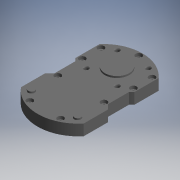
# Autodesk Inventor part: Gehaeusedeckel_Parallelform
Saved by Autodesk Inventor 2017.3 (Build 213256000, 256)
## iProperties
Part Number: Gehaeusedeckel_Parallelform
Material: Generic
Catalog Web Link: www.cadenas.de
Description: Geheausedecke-Bauteil LZ80
Vendor: ROSEKRIEGER
Document SubType Name: Modeling
Designer: partserver
Manufacturer: ROSEKRIEGER
Mass: 369.888 g
Surface Area: 551.39 cm^2
Volume: 369.888 cm^3
Density: 1 g/cm^3
Appearance: PSOLRGB-128-128-128
Category: PARTsolutions
Company: ROSEKRIEGER
Title: Gehaeusedeckel_Parallelform
Author: Cadenas PARTsolutions
Comments: Bauteil LZ80
PSOL_IDENT_0: {$CADENAS_DATA\23d-libs\rose_krieger\linearkomponenten\pool_lineartechnik\_hubsaeule_zyliinder\elekt
PSOL_IDENT_1: rozylinder\elekzyl_lz80\lz80_gehaeusedeckel.prj},192 {VTYP=3D},{NB=Gehaeusedeckel_Parallelform},{LIN
PSOL_IDENT_2: A=Gehaeusedeckel_Parallelform},{NN=Geheausedecke},{DATE=12.11.2020 14:43:35},{GEOMDATE=06.12.2006},{
PSOL_IDENT_3: VERSION=},{LINEID=10},{WBVAR=},{WBNUMERIC=}  {NB=Gehaeusedeckel_Parallelform},{LINA=Gehaeusedeckel_P
PSOL_IDENT_4: arallelform},{KT=DUMMY},{IDNR=},{ARTIKEL=Gehaeusedeckel_Parallelform},{DECKELBR1=107.310},{DECKELBR2=
PSOL_IDENT_5: 114.310},{DECKELBR3=97.310},{KONTRA1=71.450},{KONTRA2=74.100},{ABKONTRA2=25.250},{ABKONTRA1=25.240},
PSOL_IDENT_6: {ACHSAB=95.760},{HOEHE=20.000},{FUSSGROSS=44.500},{FUSSKLEIN=12.000},{FUSSKLHOE=3.000},{FUSSGRHOE=3.
PSOL_IDENT_7: 000},{ABFUSKL=18.000},{BREITFUSKL=84.000},{BEFBO1=7.450},{ABBEFBO1=56.500},{TIEFBEFBO1=20.500},{SENK
PSOL_IDENT_8: DURCH=9.500},{FASE=1.500},{SENKDURCH1=11.200},{SENKDURCH2=6.400},{SENKTIEF1=5.500},{ABSENK3U4=93.000
PSOL_IDENT_9: },{ABSENK1=84.000},{ABSENK2=56.000},{ABSENK5=39.500},{SENKAB4=113.000},{SENKAB3=79.000},{SENKAB1=30.
PSOL_IDENT_10: 000},{SENKAB2=35.000}
NB: Gehaeusedeckel_Parallelform
NN: Geheausedecke
NT: Bauteil LZ80
NBSYN: $ARTIKEL.
LINA: Gehaeusedeckel_Parallelform
CATALOG: RK Rose+Krieger
ARTIKEL: Gehaeusedeckel_Parallelform
DECKELBR1: 107.31
DECKELBR2: 114.31
DECKELBR3: 97.31
KONTRA1: 71.45
KONTRA2: 74.1
ABKONTRA2: 25.25
ABKONTRA1: 25.24
ACHSAB: 95.76
HOEHE: 20
FUSSGROSS: 44.5
FUSSKLEIN: 12
FUSSKLHOE: 3
FUSSGRHOE: 3
ABFUSKL: 18
BREITFUSKL: 84
BEFBO1: 7.45
ABBEFBO1: 56.5
TIEFBEFBO1: 20.5
SENKDURCH: 9.5
FASE: 1.5
SENKDURCH1: 11.2
SENKDURCH2: 6.4
SENKTIEF1: 5.5
ABSENK3U4: 93
ABSENK1: 84
ABSENK2: 56
ABSENK5: 39.5
SENKAB4: 113
SENKAB3: 79
SENKAB1: 30
SENKAB2: 35
SUPPLIER: ROSEKRIEGER
ARTICLENO: Gehaeusedeckel_Parallelform
BOMINFO: Gehaeusedeckel_Parallelform
CREATOR: CADENAS GmbH
Autodesk Inventor part; units mm, degrees
ref_plane "YZ Plane" through (0, 0, 0) normal (1, 0, 0) x (0, 1, 0)
ref_plane "XZ Plane" through (0, 0, 0) normal (0, 1, 0) x (-1, 0, 0)
ref_plane "XY Plane" through (0, 0, 0) normal (0, 0, 1) x (1, 0, 0)
sketch "Skizze_1" plane through (0, 0, 0) normal (0, 0, 1) x (1, 0, 0)
  line L0 (-57.155, -25.9695) -> (-57.155, -69.7905)
  arc A0 (-57.155, -69.7905) -> (57.155, -69.7905) centre (0, -22.63) ccw
  line L1 (57.155, -69.7905) -> (57.155, -25.9695)
  arc A1 (57.155, -25.9695) -> (48.655, -17.2417) centre (0, -73.13) ccw
  line L2 (48.655, -17.2417) -> (48.655, 20.7961)
  arc A2 (48.655, 20.7961) -> (53.655, 25.9369) centre (0, 73.12) ccw
  line L3 (53.655, 25.9369) -> (53.655, 69.8231)
  arc A3 (53.655, 69.8231) -> (-53.655, 69.8231) centre (0, 22.64) ccw
  line L4 (-53.655, 69.8231) -> (-53.655, 25.9369)
  arc A4 (-53.655, 25.9369) -> (-48.655, 20.7961) centre (0, 73.12) ccw
  line L5 (-48.655, 20.7961) -> (-48.655, -17.2417)
  arc A5 (-48.655, -17.2417) -> (-57.155, -25.9695) centre (0, -73.13) ccw
  constraints: 12 end point, 12 point on circle, 6 centre point
extrude "Extrusion1" add sketch "Skizze_1" along normal blind 20
sketch "Skizze_2" plane through (0, 0, 0) normal (0, 0, 1) x (1, 0, 0)
  circle A0 centre (0, 47.88) radius 22.25
  constraints: 1 centre point
extrude "Extrusion2" add sketch "Skizze_2" against normal blind 3
sketch "Skizze_3" plane through (0, 0, 0) normal (0, 0, 1) x (1, 0, 0)
  circle A0 centre (42, -65.88) radius 6
  constraints: 1 centre point
extrude "Extrusion3" add sketch "Skizze_3" against normal blind 3
sketch "Skizze_4" plane through (0, 0, 0) normal (0, 0, 1) x (1, 0, 0)
  circle A0 centre (-42, -65.88) radius 6
  constraints: 1 centre point
extrude "Extrusion4" add sketch "Skizze_4" against normal blind 3
sketch "Skizze_6" plane through (0, 0, 20) normal (0, 0, 1) x (1, 0, 0)
  circle A0 centre (28.25, 76.13) radius 4.75
  constraints: 1 centre point
extrude "Extrusion5" add sketch "Skizze_6" along normal blind 3
pattern_linear "Rectangular Pattern1" count 2 spacing 56.5 along (-1, 0, 0) count 2 spacing 56.5 along (0, -1, 0) of "Extrusion5"
sketch "Sketch6" plane through (0, 0, 0) normal (0, 0, -1) x (-1, 0, 0)
  point P0 (-28.25, 19.63)
hole "Hole1" at (28.25, 19.63, 0) direction (0, 0, 1) diameter 7.45 depth 20.5 countersink diameter 9.5 countersink angle 68.692
sketch "Sketch7" plane through (0, 0, 0) normal (0, 0, -1) x (-1, 0, 0)
  point P0 (-28.25, 76.13)
hole "Hole2" at (28.25, 76.13, 0) direction (0, 0, 1) diameter 7.45 depth 20.5 countersink diameter 9.5 countersink angle 68.692
sketch "Sketch8" plane through (0, 0, 0) normal (0, 0, -1) x (-1, 0, 0)
  point P0 (28.25, 19.63)
hole "Hole3" at (-28.25, 19.63, 0) direction (0, 0, 1) diameter 7.45 depth 20.5 countersink diameter 9.5 countersink angle 68.692
sketch "Sketch9" plane through (0, 0, 0) normal (0, 0, -1) x (-1, 0, 0)
  point P0 (28.25, 76.13)
hole "Hole4" at (-28.25, 76.13, 0) direction (0, 0, 1) diameter 7.45 depth 20.5 countersink diameter 9.5 countersink angle 68.692
sketch "Sketch10" plane through (0, 0, 0) normal (0, 0, -1) x (-1, 0, 0)
  point P0 (0, 87.38)
hole "Hole5" at (0, 87.38, 0) direction (0, 0, 1) diameter 6.4 depth 20 counterbore diameter 11.2 counterbore depth 5.5
sketch "Sketch11" plane through (0, 0, 0) normal (0, 0, -1) x (-1, 0, 0)
  point P0 (46.5, 65.12)
hole "Hole6" at (-46.5, 65.12, 0) direction (0, 0, 1) diameter 6.4 depth 20 counterbore diameter 11.2 counterbore depth 5.5
sketch "Sketch12" plane through (0, 0, 0) normal (0, 0, -1) x (-1, 0, 0)
  point P0 (46.5, 31.12)
hole "Hole7" at (-46.5, 31.12, 0) direction (0, 0, 1) diameter 6.4 depth 20 counterbore diameter 11.2 counterbore depth 5.5
sketch "Sketch13" plane through (0, 0, 0) normal (0, 0, -1) x (-1, 0, 0)
  point P0 (42, -17.88)
hole "Hole8" at (-42, -17.88, 0) direction (0, 0, 1) diameter 6.4 depth 20 counterbore diameter 11.2 counterbore depth 5.5
sketch "Sketch14" plane through (0, 0, 0) normal (0, 0, -1) x (-1, 0, 0)
  point P0 (28, -82.88)
hole "Hole9" at (-28, -82.88, 0) direction (0, 0, 1) diameter 6.4 depth 20 counterbore diameter 11.2 counterbore depth 5.5
sketch "Sketch15" plane through (0, 0, 0) normal (0, 0, -1) x (-1, 0, 0)
  point P0 (-46.5, 65.12)
hole "Hole10" at (46.5, 65.12, 0) direction (0, 0, 1) diameter 6.4 depth 20 counterbore diameter 11.2 counterbore depth 5.5
sketch "Sketch16" plane through (0, 0, 0) normal (0, 0, -1) x (-1, 0, 0)
  point P0 (-46.5, 31.12)
hole "Hole11" at (46.5, 31.12, 0) direction (0, 0, 1) diameter 6.4 depth 20 counterbore diameter 11.2 counterbore depth 5.5
sketch "Sketch17" plane through (0, 0, 0) normal (0, 0, -1) x (-1, 0, 0)
  point P0 (-42, -17.88)
hole "Hole12" at (42, -17.88, 0) direction (0, 0, 1) diameter 6.4 depth 20 counterbore diameter 11.2 counterbore depth 5.5
sketch "Sketch18" plane through (0, 0, 0) normal (0, 0, -1) x (-1, 0, 0)
  point P0 (-28, -82.88)
hole "Hole13" at (28, -82.88, 0) direction (0, 0, 1) diameter 6.4 depth 20 counterbore diameter 11.2 counterbore depth 5.5
ref_plane "EPDOPPENNUT_XY" through (0, 47.88, 20) normal (0, 0, 1) x (1, 0, 0)
ref_plane "EPDOPPENNUT_YZ" through (0, 47.88, 20) normal (1, 0, 0) x (0, 1, 0)
ref_plane "EPDOPPENNUT_ZX" through (0, 47.88, 20) normal (0, 1, 0) x (0, 0, 1)
ref_plane "EPFUNKTIONPR_XY" through (0, -47.88, 20) normal (0, 0, 1) x (1, 0, 0)
ref_plane "EPFUNKTIONPR_YZ" through (0, -47.88, 20) normal (1, 0, 0) x (0, 1, 0)
ref_plane "EPFUNKTIONPR_ZX" through (0, -47.88, 20) normal (0, 1, 0) x (0, 0, 1)
ref_plane "EPZYL1_XY" through (46.5, 65.12, 5.5) normal (0, 0, 1) x (1, 0, 0)
ref_plane "EPZYL1_YZ" through (46.5, 65.12, 5.5) normal (1, 0, 0) x (0, 1, 0)
ref_plane "EPZYL1_ZX" through (46.5, 65.12, 5.5) normal (0, 1, 0) x (0, 0, 1)
ref_plane "EPZYL2_XY" through (-46.5, 65.12, 5.5) normal (0, 0, 1) x (1, 0, 0)
ref_plane "EPZYL2_YZ" through (-46.5, 65.12, 5.5) normal (1, 0, 0) x (0, 1, 0)
ref_plane "EPZYL2_ZX" through (-46.5, 65.12, 5.5) normal (0, 1, 0) x (0, 0, 1)
ref_plane "EPZYL3_XY" through (46.5, 31.12, 5.5) normal (0, 0, 1) x (1, 0, 0)
ref_plane "EPZYL3_YZ" through (46.5, 31.12, 5.5) normal (1, 0, 0) x (0, 1, 0)
ref_plane "EPZYL3_ZX" through (46.5, 31.12, 5.5) normal (0, 1, 0) x (0, 0, 1)
ref_plane "EPZYL4_XY" through (-46.5, 31.12, 5.5) normal (0, 0, 1) x (1, 0, 0)
ref_plane "EPZYL4_YZ" through (-46.5, 31.12, 5.5) normal (1, 0, 0) x (0, 1, 0)
ref_plane "EPZYL4_ZX" through (-46.5, 31.12, 5.5) normal (0, 1, 0) x (0, 0, 1)
ref_plane "EPZYL5_XY" through (42, -17.88, 5.5) normal (0, 0, 1) x (1, 0, 0)
ref_plane "EPZYL5_YZ" through (42, -17.88, 5.5) normal (1, 0, 0) x (0, 1, 0)
ref_plane "EPZYL5_ZX" through (42, -17.88, 5.5) normal (0, 1, 0) x (0, 0, 1)
ref_plane "EPZYL6_XY" through (-42, -17.88, 5.5) normal (0, 0, 1) x (1, 0, 0)
ref_plane "EPZYL6_YZ" through (-42, -17.88, 5.5) normal (1, 0, 0) x (0, 1, 0)
ref_plane "EPZYL6_ZX" through (-42, -17.88, 5.5) normal (0, 1, 0) x (0, 0, 1)
ref_plane "EPZYL7_XY" through (28, -82.88, 5.5) normal (0, 0, 1) x (1, 0, 0)
ref_plane "EPZYL7_YZ" through (28, -82.88, 5.5) normal (1, 0, 0) x (0, 1, 0)
ref_plane "EPZYL7_ZX" through (28, -82.88, 5.5) normal (0, 1, 0) x (0, 0, 1)
ref_plane "EPZYL8_XY" through (-28, -82.88, 5.5) normal (0, 0, 1) x (1, 0, 0)
ref_plane "EPZYL8_YZ" through (-28, -82.88, 5.5) normal (1, 0, 0) x (0, 1, 0)
ref_plane "EPZYL8_ZX" through (-28, -82.88, 5.5) normal (0, 1, 0) x (0, 0, 1)
ref_plane "EPZYL9_XY" through (0, 87.38, 5.5) normal (0, 0, 1) x (1, 0, 0)
ref_plane "EPZYL9_YZ" through (0, 87.38, 5.5) normal (1, 0, 0) x (0, 1, 0)
ref_plane "EPZYL9_ZX" through (0, 87.38, 5.5) normal (0, 1, 0) x (0, 0, 1)
body "Solid1"
